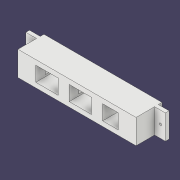
# Autodesk Inventor part: BP011
Saved by Autodesk Inventor 2017 SP1 (Build 210196100, 196)
## iProperties
Created: 2018-06-18
Part Number: BP011
Material: ABS Plastic
Document SubType Name: Modeling
Designer: Zach
Density: 1.06 g/cm^3
Appearance: CR White
Author: Zach
Autodesk Inventor part; units mm, degrees
ref_plane "YZ Plane" through (0, 0, 0) normal (1, 0, 0) x (0, 1, 0)
ref_plane "XZ Plane" through (0, 0, 0) normal (0, 1, 0) x (-1, 0, 0)
ref_plane "XY Plane" through (0, 0, 0) normal (0, 0, 1) x (1, 0, 0)
sketch "Sketch1" plane through (0, 0, 0) normal (0, 0, 1) x (1, 0, 0)
  line L0 (0, 0) -> (190, 0)
  line L1 (190, 0) -> (190, 35)
  line L2 (190, 35) -> (0, 35)
  line L3 (0, 35) -> (0, 0)
  circle A0 centre (7.5, 17.5) radius 1.5
  circle A1 centre (182.5, 17.5) radius 1.5
  point P0 (0, 17.5)
  dimension "d0" = 190
  dimension "d1" = 35
  dimension "d2" = 3
  dimension "d3" = 7.5
  dimension "d4" = 3
  dimension "d5" = 7.5
  constraints: 8 end point, 2 centre point, 2 horizontal alignment, 2 parallel, 1 horizontal, 1 midpoint, 1 perpendicular
  measures "d0" distance of L2.end L1.end
  measures "d1" distance of L1.end L0.end
  measures "d2" diameter of A0
  measures "d3" distance from line of L3 A0.centre
  measures "d4" diameter of A1
  measures "d5" distance from line of L1 A1.centre
extrude "Extrusion1" add sketch "Sketch1" along normal blind 5
sketch "Sketch2" plane through (0, 0, 0) normal (0, 0, -1) x (-1, 0, 0)
  line L0 (0, 0) -> (-190, 0) projected
  line L1 (-190, 35) -> (0, 35) projected
  line L2 (-15.5, 0) -> (-174.5, 0)
  line L3 (-174.5, 0) -> (-174.5, 35)
  line L4 (-174.5, 35) -> (-15.5, 35)
  line L5 (-15.5, 35) -> (-15.5, 0)
  point P0 (-95, 0)
  dimension "d8" = 159
  constraints: 8 end point, 2 midpoint, 2 parallel, 2 point on line, 1 horizontal, 1 perpendicular
  measures "d8" distance between parallel lines of L5 L3
extrude "Extrusion2" add sketch "Sketch2" along normal blind 5
sketch "Sketch3" plane through (0, 0, 5) normal (0, 0, 1) x (1, 0, 0)
  circle A0 centre (182.5, 17.5) radius 1.5 projected
  circle A1 centre (7.5, 17.5) radius 1.5 projected
  line L0 (0, 0) -> (190, 0) projected
  line L1 (190, 0) -> (190, 35) projected
  line L2 (190, 35) -> (0, 35) projected
  line L3 (0, 35) -> (0, 0) projected
  line L4 (1, 34) -> (189, 34)
  line L5 (189, 34) -> (189, 1)
  line L6 (189, 1) -> (1, 1)
  line L7 (1, 1) -> (1, 34)
  dimension "d11" = 1
  constraints: 8 end point, 3 other
  measures "d11" distance between parallel lines of L2 L4
extrude "Extrusion3" cut sketch "Sketch3" against normal through all contours L3 L2 L1 L0
sketch "Sketch4" plane through (0, 0, 5) normal (0, 0, 1) x (1, 0, 0)
  line L0 (39.5, 27.5) -> (69.5, 27.5)
  line L1 (69.5, 27.5) -> (69.5, 7.5)
  line L2 (69.5, 7.5) -> (39.5, 7.5)
  line L3 (39.5, 7.5) -> (39.5, 27.5)
  line L4 (84.5, 27.5) -> (114.5, 27.5)
  line L5 (114.5, 27.5) -> (114.5, 7.5)
  line L6 (114.5, 7.5) -> (84.5, 7.5)
  line L7 (84.5, 7.5) -> (84.5, 27.5)
  line L8 (129.5, 27.5) -> (150.5, 27.5)
  line L9 (150.5, 27.5) -> (150.5, 7.5)
  line L10 (150.5, 7.5) -> (129.5, 7.5)
  line L11 (129.5, 7.5) -> (129.5, 27.5)
  line L12 (39.5, 17.5) -> (150.5, 17.5) construction
  line L13 (189, 34) -> (1, 34) projected
  circle A0 centre (7.5, 17.5) radius 1.5 projected
  point P0 (0, 0)
  point P1 (95, 17.5)
  point P2 (95, 34)
  point P3 (114.5, 17.5)
  dimension "d14" = 30
  dimension "d15" = 20
  dimension "d16" = 30
  dimension "d17" = 20
  dimension "d18" = 21
  dimension "d19" = 20
  dimension "d20" = 15
  dimension "d21" = 15
  constraints: 26 end point, 6 parallel, 5 midpoint, 3 horizontal, 3 perpendicular, 2 horizontal alignment, 1 point on line, 1 vertical alignment
  measures "d14" distance of L1.end L2.end
  measures "d15" distance of L0.end L1.end
  measures "d16" distance of L5.end L6.end
  measures "d17" distance of L4.end L5.end
  measures "d18" distance of L9.end L10.end
  measures "d19" distance of L8.end L9.end
  measures "d20" distance between parallel lines of L1 L7
  measures "d21" distance between parallel lines of L11 L5
extrude "Extrusion4" cut sketch "Sketch4" against normal through all contours L0 L1 L2 L3 | L4 L5 L6 L7 | L8 L9 L10 L11
sketch "Sketch5" plane through (0, 0, 5) normal (0, 0, 1) x (1, 0, 0)
  line L0 (39.5, 27.5) -> (39.5, 7.5) projected
  line L1 (39.5, 7.5) -> (69.5, 7.5) projected
  line L2 (69.5, 7.5) -> (69.5, 27.5) projected
  line L3 (69.5, 27.5) -> (39.5, 27.5) projected
  line L4 (129.5, 27.5) -> (129.5, 7.5) projected
  line L5 (129.5, 7.5) -> (150.5, 7.5) projected
  line L6 (150.5, 7.5) -> (150.5, 27.5) projected
  line L7 (150.5, 27.5) -> (129.5, 27.5) projected
  line L8 (84.5, 27.5) -> (84.5, 7.5) projected
  line L9 (84.5, 7.5) -> (114.5, 7.5) projected
  line L10 (114.5, 7.5) -> (114.5, 27.5) projected
  line L11 (114.5, 27.5) -> (84.5, 27.5) projected
  line L12 (174.5, 1) -> (15.5, 1) projected
  line L13 (15.5, 1) -> (15.5, 34) projected
  line L14 (15.5, 34) -> (174.5, 34) projected
  line L15 (174.5, 34) -> (174.5, 1) projected
  point P0 (0, 0)
extrude "Extrusion5" add sketch "Sketch5" along normal blind 25
sketch "Sketch6" plane through (0, 0, -5) normal (0, 0, -1) x (-1, 0, 0)
  line L0 (-69.5, 27.5) -> (-39.5, 27.5) projected
  line L1 (-39.5, 27.5) -> (-39.5, 7.5) projected
  line L2 (-69.5, 7.5) -> (-69.5, 27.5) projected
  line L3 (-84.5, 27.5) -> (-84.5, 7.5) projected
  line L4 (-114.5, 27.5) -> (-84.5, 27.5) projected
  line L5 (-114.5, 7.5) -> (-114.5, 27.5) projected
  line L6 (-39.5, 25) -> (-34.5, 25)
  line L7 (-34.5, 25) -> (-34.5, 10)
  line L8 (-34.5, 10) -> (-39.5, 10)
  line L9 (-39.5, 10) -> (-39.5, 25)
  line L10 (-69.5, 25) -> (-74.5, 25)
  line L11 (-74.5, 25) -> (-74.5, 10)
  line L12 (-74.5, 10) -> (-69.5, 10)
  line L13 (-69.5, 10) -> (-69.5, 25)
  line L14 (-84.5, 25) -> (-79.5, 25)
  line L15 (-79.5, 25) -> (-79.5, 10)
  line L16 (-79.5, 10) -> (-84.5, 10)
  line L17 (-84.5, 10) -> (-84.5, 25)
  line L18 (-114.5, 25) -> (-119.5, 25)
  line L19 (-119.5, 25) -> (-119.5, 10)
  line L20 (-119.5, 10) -> (-114.5, 10)
  line L21 (-114.5, 10) -> (-114.5, 25)
  point P0 (0, 0)
  point P1 (-39.5, 17.5)
  dimension "d26" = 15
  dimension "d27" = 5
  dimension "d28" = 5
  dimension "d29" = 5
  dimension "d30" = 5
  constraints: 32 end point, 8 parallel, 6 horizontal alignment, 4 horizontal, 4 perpendicular, 4 point on line, 2 midpoint
  measures "d26" distance of L6.end L7.end
  measures "d27" distance of L6.start L6.end
  measures "d28" distance of L10.start L10.end
  measures "d29" distance of L14.start L14.end
  measures "d30" distance of L18.start L18.end
extrude "Extrusion6" cut sketch "Sketch6" against normal blind 22
body "Solid1"
